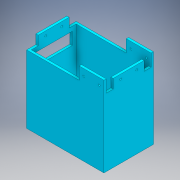
# Autodesk Inventor part: Main Part
Saved by Autodesk Inventor 2017 (Build 210142000, 142)
## iProperties
Created: 2017-12-22
Part Number: Main Part
Material: Generic
Document SubType Name: Modeling
Designer: Dharsan
Density: 1 g/cm^3
Appearance: Default
Author: Dharsan
Autodesk Inventor part; units mm, degrees
ref_plane "XY Plane" through (0, 0, 0) normal (0, 0, 1) x (1, 0, 0)
sketch "Sketch1" plane through (0, 0, 0) normal (0, 0, 1) x (1, 0, 0)
  line L0 (0, 0) -> (125, 0)
  line L1 (125, 0) -> (125, 80)
  line L2 (125, 80) -> (0, 80)
  line L3 (0, 80) -> (0, 0)
  dimension "d0" = 125
  dimension "d1" = 80
  constraints: 8 end point, 2 horizontal, 2 perpendicular
  measures "d0" distance of L0.start L0.end
  measures "d1" distance of L0.end L1.end
extrude "Extrusion1" add sketch "Sketch1" along normal blind 110
shell "Shell1" thickness 3.75 removed faces 1 at (83.3333, 26.6667, 110)
sketch "Sketch2" plane through (0, 0, 0) normal (0, 0, -1) x (-1, 0, 0)
  line L0 (0, 80) -> (0, 0) projected
  line L1 (-125, 80) -> (0, 80) projected
  line L2 (0, 0) -> (-125, 0) projected
  line L3 (-125, 0) -> (-125, 80) projected
  circle A0 centre (-118, 27.634) radius 1.5
  circle A1 centre (-118, 45.733) radius 1.5
  circle A2 centre (-79.9, 7) radius 1.5
  circle A3 centre (-61.929, 7) radius 1.5
  line L4 (-62.4, 53.8768) -> (-79.9, 53.8768)
  line L5 (-79.9, 53.8768) -> (-79.9, 20.8768)
  line L6 (-79.9, 20.8768) -> (-62.4, 20.8768)
  line L7 (-62.4, 20.8768) -> (-62.4, 53.8768)
  dimension "d22" = 3
  dimension "d23" = 3
  dimension "d24" = 7
  dimension "d25" = 7
  dimension "d26" = 27.634
  dimension "d46" = 45.733
  dimension "d77" = 3
  dimension "d78" = 3
  dimension "d79" = 7
  dimension "d80" = 7
  dimension "d81" = 45.1
  dimension "d82" = 63.071
  dimension "d83" = 45.1
  dimension "d84" = 20.8768
  dimension "d85" = 33
  dimension "d86" = 17.5
  constraints: 8 end point, 4 centre point, 2 parallel, 1 horizontal, 1 perpendicular
  measures "d22" diameter of A0
  measures "d23" diameter of A1
  measures "d24" distance from line of L3 A1.centre
  measures "d25" distance from line of L3 A0.centre
  measures "d26" distance from line of L2 A0.centre
  measures "d46" distance from line of L2 A1.centre
  measures "d77" diameter of A2
  measures "d78" diameter of A3
  measures "d79" distance from line of L2 A3.centre
  measures "d80" distance from line of L2 A2.centre
  measures "d81" distance from line of L3 A2.centre
  measures "d82" distance from line of L3 A3.centre
  measures "d83" distance between parallel lines of L3 L5
  measures "d84" distance between parallel lines of L2 L6
  measures "d85" distance of L6.end L4.start
  measures "d86" distance of L4.start L4.end
extrude "Extrusion6" cut sketch "Sketch2" against normal blind 20 contours A0 | A1 | A2 | A3 | L7 L6 L5 L4
sketch "Sketch6" plane through (0, 80, 0) normal (0, 1, 0) x (1, 0, 0)
  line L0 (0, -110) -> (125, -110) projected
  line L1 (125, -110) -> (85, -110)
  line L2 (85, -110) -> (85, -130)
  line L3 (85, -130) -> (125, -130)
  line L4 (125, -130) -> (125, -110)
  point P0 (0, 0)
  dimension "d53" = 40
  dimension "d54" = 20
  constraints: 8 end point, 2 parallel, 1 horizontal, 1 perpendicular
  measures "d53" distance of L3.end L2.end
  measures "d54" distance of L2.end L1.end
extrude "Extrusion8" add sketch "Sketch6" against normal blind 3.75
ref_plane "Work Plane1" through (0, 40, 0) normal (0, 1, 0) x (-1, 0, 0)
mirror "Mirror1" about plane through (0, 40, 0) normal (0, 1, 0) of "Extrusion8"
sketch "Sketch7" plane through (0, 0, 0) normal (-1, 0, 0) x (0, 0, 1)
  line L0 (110, 3.75) -> (110, 76.25) projected
  line L1 (110, 15) -> (125, 15)
  line L2 (125, 15) -> (125, 65)
  line L3 (125, 65) -> (110, 65)
  line L4 (110, 65) -> (110, 15)
  line L5 (130, 76.25) -> (110, 76.25) projected
  line L6 (130, 3.75) -> (110, 3.75) projected
  point P0 (0, 0)
  dimension "d58" = 15
  dimension "d59" = 50
  dimension "d60" = 11.25
  dimension "d61" = 11.25
  constraints: 8 end point, 2 parallel, 1 horizontal, 1 perpendicular, 1 point on line
  measures "d58" distance of L3.end L2.end
  measures "d59" distance of L1.end L2.end
  measures "d60" distance between parallel lines of L5 L3
  measures "d61" distance between parallel lines of L1 L6
extrude "Extrusion9" add sketch "Sketch7" against normal blind 3.75
ref_plane "Work Plane2" through (62.5, 0, 0) normal (1, 0, 0) x (0, 1, 0)
mirror "Mirror2" about plane through (62.5, 0, 0) normal (1, 0, 0) of "Extrusion9"
sketch "Sketch8" plane through (0, 0, 0) normal (-1, 0, 0) x (0, 0, 1)
  line L0 (103, 70) -> (83, 70)
  line L1 (83, 70) -> (83, 10)
  line L2 (83, 10) -> (103, 10)
  line L3 (103, 10) -> (103, 70)
  line L4 (110, 3.75) -> (110, 15) projected
  line L5 (0, 0) -> (110, 0) projected
  line L6 (0, 80) -> (110, 80) projected
  dimension "d70" = 20
  dimension "d71" = 60
  dimension "d72" = 7
  dimension "d73" = 10
  dimension "d74" = 10
  constraints: 8 end point, 2 parallel, 1 horizontal, 1 perpendicular
  measures "d70" distance of L2.end L1.end
  measures "d71" distance of L1.end L0.end
  measures "d72" distance between parallel lines of L4 L3
  measures "d73" distance between parallel lines of L5 L2
  measures "d74" distance between parallel lines of L6 L0
extrude "Extrusion11" cut sketch "Sketch8" against normal blind 10
sketch "Sketch9" plane through (0, 0, 0) normal (-1, 0, 0) x (0, 0, 1)
  circle A0 centre (118, 53) radius 1.5
  circle A1 centre (118, 27) radius 1.5
  line L0 (110, 15) -> (125, 15) projected
  line L1 (125, 15) -> (125, 65) projected
  line L2 (125, 65) -> (110, 65) projected
  point P0 (0, 0)
  dimension "d87" = 3
  dimension "d88" = 3
  dimension "d89" = 12
  dimension "d90" = 7
  dimension "d91" = 12
  dimension "d92" = 7
  constraints: 2 centre point
  measures "d87" diameter of A0
  measures "d88" diameter of A1
  measures "d89" distance from line of L0 A1.centre
  measures "d90" distance from line of L1 A1.centre
  measures "d91" distance from line of L2 A0.centre
  measures "d92" distance from line of L1 A0.centre
extrude "Extrusion12" cut sketch "Sketch9" against normal blind 200
sketch "Sketch10" plane through (0, 0, 0) normal (0, -1, 0) x (1, 0, 0)
  circle A0 centre (92.5, 119.3503) radius 1.5
  circle A1 centre (117.5, 119.3503) radius 1.5
  line L0 (125, 0) -> (125, 130) projected
  line L1 (85, 110) -> (85, 130) projected
  line L2 (85, 130) -> (125, 130) projected
  point P0 (0, 0)
  dimension "d95" = 3
  dimension "d96" = 3
  dimension "d97" = 7.5
  dimension "d98" = 7.5
  dimension "d99" = 10.6497
  dimension "d100" = 10.6497
  constraints: 2 centre point
  measures "d95" diameter of A0
  measures "d96" diameter of A1
  measures "d97" distance from line of L0 A1.centre
  measures "d98" distance from line of L1 A0.centre
  measures "d99" distance from line of L2 A0.centre
  measures "d100" distance from line of L2 A1.centre
extrude "Extrusion13" cut sketch "Sketch10" against normal blind 100
body "Solid1"
